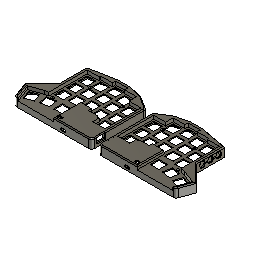
top_3x5_3 (Autodesk Fusion 360 design; units mm, degrees)
Autodesk Fusion 360 part; units mm, degrees
note: some values were not read from the file. Chosen so that the rebuilt part matches the saved one: which pieces of a blend or face edit are solid. Set by a fixed rule: which sketch regions a step uses.
sketch "case_plate_3x5_3" plane through (0, 0, 0) normal (0, 0, 1) x (1, 0, 0)
  line L0 (28.1017, -18.5688) -> (8.5, -30.9488)
  line L1 (8.5, -30.9488) -> (8.5, -112.72)
  line L2 (8.5, -112.72) -> (126.2948, -112.72)
  line L3 (133.9348, -91.7293) -> (107.5, -65.3353)
  line L4 (107.5, -65.3353) -> (107.5, -21.174)
  line L5 (126.2948, -112.72) -> (133.9348, -91.7293)
  line L6 (107.5, -21.174) -> (67.6888, -13.518)
  line L7 (67.6888, -13.518) -> (67.5953, -13.5)
  line L8 (67.5953, -13.5) -> (48.3769, -13.5)
  line L9 (48.3769, -13.5) -> (28.1017, -18.5688)
  line L10 (137.4081, -90.9579) -> (110.5, -64.0913)
  line L11 (5.5, -115.72) -> (128.3954, -115.72)
  line L12 (5.5, -29.2953) -> (5.5, -115.72)
  line L13 (110.5, -64.0913) -> (110.5, -18.6959)
  line L14 (26.9069, -15.7752) -> (5.5, -29.2953)
  line L15 (128.3954, -115.72) -> (137.4081, -90.9579)
  line L16 (110.5, -18.6959) -> (67.8811, -10.5)
  line L17 (48.0076, -10.5) -> (26.9069, -15.7752)
  line L18 (67.8811, -10.5) -> (48.0076, -10.5)
  line L19 (135.3241, -91.4207) -> (108.7, -64.8377)
  line L20 (108.7, -64.8377) -> (108.7, -20.1828)
  line L21 (127.135, -113.92) -> (135.3241, -91.4207)
  line L22 (48.2292, -12.3) -> (27.6238, -17.4513)
  line L23 (67.7096, -12.3) -> (48.2292, -12.3)
  line L24 (108.7, -20.1828) -> (67.7096, -12.3)
  line L25 (27.6238, -17.4513) -> (7.3, -30.2874)
  line L26 (7.3, -30.2874) -> (7.3, -113.92)
  line L27 (7.3, -113.92) -> (127.135, -113.92)
  line L28 (27.3848, -16.8926) -> (6.7, -29.9567)
  line L29 (136.0188, -91.2664) -> (109.3, -64.5889)
  line L30 (48.1553, -11.7) -> (27.3848, -16.8926)
  line L31 (6.7, -29.9567) -> (6.7, -114.52)
  line L32 (127.5552, -114.52) -> (136.0188, -91.2664)
  line L33 (67.7668, -11.7) -> (48.1553, -11.7)
  line L34 (109.3, -64.5889) -> (109.3, -19.6872)
  line L35 (68.0288, -11.7504) -> (67.7668, -11.7)
  line L36 (6.7, -114.52) -> (127.5552, -114.52)
  line L37 (109.3, -19.6872) -> (68.0288, -11.7504)
  circle A0 centre (32, -39.5) radius 2.2
  circle A1 centre (84, -39.5) radius 2.2
  circle A2 centre (100.1356, -83.3241) radius 2.2
  line L38 (43.5, -109.61) -> (43.5, -91.61)
  line L39 (10.5, -91.61) -> (10.5, -109.61)
  line L40 (43.5, -91.61) -> (10.5, -91.61)
  line L41 (10.5, -109.61) -> (43.5, -109.61)
  line L42 (47.025, -106.99) -> (47.025, -112.84)
  line L43 (55.825, -112.84) -> (55.825, -106.99)
  line L44 (55.825, -106.99) -> (47.025, -106.99)
  line L45 (66.825, -107.975) -> (57.825, -107.975)
  line L46 (66.825, -111.475) -> (66.825, -107.975)
  line L47 (57.825, -107.975) -> (57.825, -111.475)
  line L48 (57.825, -111.475) -> (66.825, -111.475)
  line L49 (122.6064, -82.1718) -> (114.8282, -74.3936)
  line L50 (114.8282, -74.3936) -> (108.3936, -80.8282)
  line L51 (108.3936, -80.8282) -> (110.7585, -83.1932)
  line L52 (118.9049, -85.8732) -> (122.6064, -82.1718)
  line L53 (43.2, -88.45) -> (43.2, -79.55)
  line L54 (43.2, -79.55) -> (34.7125, -79.55)
  line L55 (34.6, -79.6909) -> (34.6, -88.45)
  line L56 (34.6, -88.45) -> (43.2, -88.45)
  line L57 (27, -87) -> (27, -73)
  line L58 (13, -73) -> (13, -87)
  line L59 (13, -87) -> (27, -87)
  line L60 (27, -73) -> (13, -73)
  line L61 (27, -54) -> (13, -54)
  line L62 (27, -68) -> (27, -54)
  line L63 (13, -68) -> (27, -68)
  line L64 (13, -54) -> (13, -68)
  line L65 (13, -49) -> (27, -49)
  line L66 (13, -35) -> (13, -49)
  line L67 (27, -35) -> (13, -35)
  line L68 (27, -49) -> (27, -35)
  line L69 (32, -75) -> (46, -75)
  line L70 (46, -61) -> (32, -61)
  line L71 (32, -61) -> (32, -75)
  line L72 (46, -75) -> (46, -61)
  line L73 (32, -56) -> (46, -56)
  line L74 (46, -56) -> (46, -42)
  line L75 (32, -42) -> (32, -56)
  line L76 (46, -42) -> (32, -42)
  line L77 (46, -37) -> (46, -23)
  line L78 (32, -23) -> (32, -37)
  line L79 (32, -37) -> (46, -37)
  line L80 (46, -23) -> (32, -23)
  line L81 (65, -70) -> (65, -56)
  line L82 (65, -56) -> (51, -56)
  line L83 (51, -70) -> (65, -70)
  line L84 (51, -56) -> (51, -70)
  line L85 (51, -51) -> (65, -51)
  line L86 (65, -37) -> (51, -37)
  line L87 (65, -51) -> (65, -37)
  line L88 (51, -37) -> (51, -51)
  line L89 (51, -18) -> (51, -32)
  line L90 (65, -32) -> (65, -18)
  line L91 (65, -18) -> (51, -18)
  line L92 (51, -32) -> (65, -32)
  line L93 (84, -75) -> (84, -61)
  line L94 (70, -75) -> (84, -75)
  line L95 (84, -61) -> (70, -61)
  line L96 (70, -61) -> (70, -75)
  line L97 (84, -56) -> (84, -42)
  line L98 (70, -42) -> (70, -56)
  line L99 (70, -56) -> (84, -56)
  line L100 (84, -42) -> (70, -42)
  line L101 (70, -37) -> (84, -37)
  line L102 (70, -23) -> (70, -37)
  line L103 (84, -23) -> (70, -23)
  line L104 (84, -37) -> (84, -23)
  line L105 (89, -77.5) -> (103, -77.5)
  line L106 (103, -77.5) -> (103, -63.5)
  line L107 (103, -63.5) -> (89, -63.5)
  line L108 (89, -63.5) -> (89, -77.5)
  line L109 (89, -44.5) -> (89, -58.5)
  line L110 (103, -44.5) -> (89, -44.5)
  line L111 (89, -58.5) -> (103, -58.5)
  line L112 (103, -58.5) -> (103, -44.5)
  line L113 (89, -39.5) -> (103, -39.5)
  line L114 (89, -25.5) -> (89, -39.5)
  line L115 (103, -25.5) -> (89, -25.5)
  line L116 (103, -39.5) -> (103, -25.5)
  line L117 (84, -83.8) -> (70, -83.8)
  line L118 (70, -97.8) -> (84, -97.8)
  line L119 (70, -83.8) -> (70, -97.8)
  line L120 (84, -97.8) -> (84, -83.8)
  line L121 (90.3767, -98.3579) -> (104.164, -100.789)
  line L122 (92.8078, -84.5706) -> (90.3767, -98.3579)
  line L123 (104.164, -100.789) -> (106.5951, -87.0017)
  line L124 (106.5951, -87.0017) -> (92.8078, -84.5706)
  line L125 (123.5027, -107.234) -> (128.291, -94.0783)
  line L126 (115.1353, -89.29) -> (110.347, -102.4457)
  line L127 (110.347, -102.4457) -> (123.5027, -107.234)
  line L128 (128.291, -94.0783) -> (115.1353, -89.29)
  line L129 (8.5, -89.75) -> (29.75, -89.75)
  line L130 (29.75, -89.75) -> (29.75, -79.7)
  line L131 (10.25, -89.75) -> (10.25, -32.25)
  line L132 (29.25, -32.25) -> (10.25, -32.25)
  line L133 (48.75, -77.75) -> (48.75, -72.75)
  line L134 (48.25, -20.25) -> (29.25, -20.25)
  line L135 (29.25, -20.25) -> (29.25, -32.25)
  line L136 (48.75, -72.75) -> (67.25, -72.75)
  line L137 (67.75, -20.25) -> (67.75, -15.25)
  line L138 (67.75, -15.25) -> (48.25, -15.25)
  line L139 (48.25, -15.25) -> (48.25, -20.25)
  line L140 (67.25, -115.72) -> (67.25, -72.75)
  line L141 (86.75, -22.75) -> (86.75, -20.25)
  line L142 (86.75, -20.25) -> (67.75, -20.25)
  line L143 (105.75, -65.3353) -> (105.75, -22.75)
  line L144 (105.75, -22.75) -> (86.75, -22.75)
  line L145 (67.25, -100.55) -> (86.9722, -100.55)
  line L146 (86.9722, -100.55) -> (106.6135, -104.0133)
  line L147 (105.75, -84.0602) -> (111.608, -85.0931)
  line L148 (106.6135, -104.0133) -> (125.1463, -110.7587)
  line L149 (123.3406, -115.72) -> (131.8157, -92.4347)
  line L150 (111.7483, -85.1307) -> (133.4602, -93.0332)
  arc A3 (32, -79.7) -> (34.1857, -77.75) centre (32, -77.5) ccw
  line L151 (34.1857, -77.75) -> (48.75, -77.75)
  line L152 (107.5, -65.3353) -> (105.75, -65.3353)
  line L153 (105.75, -84.0602) -> (105.75, -65.3353)
  line L154 (8.5, -90.95) -> (30.95, -90.95)
  line L155 (35.0753, -78.95) -> (49.95, -78.95)
  line L156 (49.95, -78.95) -> (49.95, -73.95)
  line L157 (49.95, -73.95) -> (66.05, -73.95)
  line L158 (107.5, -82.5918) -> (107.5, -65.3353)
  line L159 (107.5, -82.5918) -> (110.4658, -83.1147)
  line L160 (113.7267, -83.9885) -> (133.327, -91.1224)
  line L161 (110.4658, -83.1147) -> (113.7267, -83.9885)
  line L162 (66.05, -112.72) -> (66.05, -73.95)
  line L163 (111.7483, -85.1307) -> (111.608, -85.0931)
  line L164 (32, -79.7) -> (29.75, -79.7)
  line L165 (8.5, -90.95) -> (30.95, -90.95)
  line L166 (30.95, -90.95) -> (30.95, -80.9)
  line L167 (32, -80.9) -> (30.95, -80.9)
  arc A4 (32, -80.9) -> (35.0753, -78.95) centre (32, -77.5) ccw
  line L168 (35.0753, -78.95) -> (49.95, -78.95)
  line L169 (49.95, -78.95) -> (49.95, -73.95)
  line L170 (49.95, -73.95) -> (66.05, -73.95)
  line L171 (66.05, -115.72) -> (66.05, -73.95)
  dimension "d85" = 1.2
  constraint tangent A3 L164
  constraint perpendicular L130 L164
extrude "inner-wall-down" add sketch "case_plate_3x5_3" against normal blind 6.8 contours L0 L1 L2 L3 L4 L5 L6 L7 L8 L9 L19 L20 L21 L22 L23 L24 L25 L26 L27 L149 L171 | L2 L27 L140 L171 | L2 L27 L140 L149 | L19 L20 L21 L22 L23 L24 L25 L26 L27 L28 L29 L30 L31 L32 L33 L34 L35 L36 L37 L149 L171 | L27 L36 L140 L171 | L27 L36 L140 L149 makes body 1
extrude "outer-wall-down" add sketch "case_plate_3x5_3" against normal blind 7.6 contours L10 L11 L12 L13 L14 L15 L16 L17 L18 L28 L29 L30 L31 L32 L33 L34 L35 L36 L37 L149 L171 | L11 L36 L140 L171 | L11 L36 L140 L149 bodies 1
extrude "switchplate" add sketch "case_plate_3x5_3" along normal blind 1.6 contours L129 L130 L131 L132 L133 L134 L135 L136 L137 L138 L139 L140 L141 L142 L143 L144 L145 L146 L147 L148 L149 L150 A3 L151 L153 L163 L164 | L2 L140 L145 L146 L148 L149 | L2 L27 L140 L149 | L27 L36 L140 L149 | L11 L36 L140 L149 | A0 | A1 | A2 bodies 1
extrude "raised-wall" add sketch "case_plate_3x5_3" along normal blind 7 contours L0 L1 L4 L6 L7 L8 L9 L129 L131 L132 L134 L135 L137 L138 L139 L141 L142 L143 L144 L152 | L0 L1 L2 L3 L4 L5 L6 L7 L8 L9 L19 L20 L21 L22 L23 L24 L25 L26 L27 L149 L171 | L1 L2 L45 L46 L48 L129 L130 L133 L136 L140 A3 L151 L154 L155 L156 L157 L162 L164 L165 L166 L167 A4 L168 L169 L170 L171 | L3 L5 L147 L150 L152 L153 L158 L159 L160 L161 L163 | L2 L27 L140 L171 | L45 L46 L48 L162 L171 | L19 L20 L21 L22 L23 L24 L25 L26 L27 L28 L29 L30 L31 L32 L33 L34 L35 L36 L37 L149 L171 | L27 L36 L140 L171 | L2 L5 L149 L150 | L10 L11 L12 L13 L14 L15 L16 L17 L18 L28 L29 L30 L31 L32 L33 L34 L35 L36 L37 L149 L171 | L11 L36 L140 L171 bodies 1
extrude "hollow-areas" add sketch "case_plate_3x5_3" along normal blind 1.6 from surface at 5.4 contours L1 L2 L42 L43 L44 L45 L47 L48 L53 L54 L55 L56 L154 L155 L156 L157 L162 L165 L166 L167 A4 L168 L169 L170 L171 | L2 L42 L43 L44 | L3 L49 L50 L51 L52 L158 L159 L160 L161 | L53 L54 L55 L56 A4 | L49 L50 L51 L52 L160 L161 | L45 L47 L48 L162 L171 | L38 L39 L40 L41 bodies 1
move_body "drop-to-hole-plane" bodies 1 to x (1, 0, 0) y (0, 1, 0) z (0, 0, 1) at (0, 0, -1.6)
hole "switchplate-holes" at (84, -39.5, 0) at (32, -39.5, 0) at (100.1356, -83.3241, 0) at (32, -77.5, 0) direction (0, 0, -1) diameter 2.4 end up to surface (1.6 mm away) countersink diameter 4.4 countersink angle 90 bodies 1
sketch "usb-cutout" plane through (5.5, 0, 0) normal (-1, 0, 0) x (0, -1, 0)
  line L0 (29.2953, 5.4) -> (29.2953, -9.2)
  line L1 (29.2953, -9.2) -> (115.72, -9.2)
  line L2 (115.72, -9.2) -> (115.72, 5.4)
  line L3 (115.72, 5.4) -> (29.2953, 5.4)
  line L4 (91.61, 0) -> (109.61, 0)
  line L5 (91.61, 4.2) -> (109.61, 4.2)
  line L6 (94.61, 4.2) -> (106.61, 4.2)
  line L7 (106.61, 4.2) -> (106.61, -3.8)
  line L8 (106.61, -3.8) -> (94.61, -3.8)
  line L9 (94.61, -3.8) -> (94.61, 4.2)
  point P0 (94.61, 4.2)
  point P1 (106.61, -3.8)
  dimension "d16" = 1.2
  dimension "d86" = 8
  constraint horizontal L6
  constraint vertical L7
  constraint horizontal L8
  constraint vertical L9
  constraint coincident P1 L7.end
  constraint coincident P0 L6.start
  measures "d16" distance of L3 L5
  measures "d86" distance of L5 P1
extrude "usb-cutout (1)" cut sketch "usb-cutout" against normal up to surface (3 mm away) contours L4 L5 L6 L7 L9 | L4 L7 L8 L9 bodies 1
sketch "vik-cutout" plane through (23.119, 23.1547, 0) normal (0.70656, 0.707653, 0) x (-0.707653, 0.70656, 0)
  line L0 (-161.5044, 5.4) -> (-161.5044, -9.2)
  line L1 (-161.5044, -9.2) -> (-123.48, -9.2)
  line L2 (-123.48, -9.2) -> (-123.48, 5.4)
  line L3 (-123.48, 5.4) -> (-161.5044, 5.4)
  line L4 (-144.8221, 0) -> (-133.8221, 0)
  line L5 (-144.8221, -5) -> (-133.8221, -5)
  line L6 (-142.8221, -4.5) -> (-135.8221, -4.5)
  line L7 (-135.8221, -4.5) -> (-135.8221, -5.5)
  line L8 (-135.8221, -5.5) -> (-142.8221, -5.5)
  line L9 (-142.8221, -5.5) -> (-142.8221, -4.5)
  point P0 (-142.8221, -4.5)
  point P1 (-135.8221, -5.5)
  dimension "d19" = 10.4
  constraint horizontal L6
  constraint vertical L7
  constraint horizontal L8
  constraint vertical L9
  constraint coincident P1 L7.end
  constraint coincident P0 L6.start
  measures "d19" distance of L3 L5
extrude "vik-cutout (1)" cut sketch "vik-cutout" against normal up to surface (3 mm away) contours L5 L6 L7 L9 | L5 L7 L8 L9 bodies 1
sketch "rst-cutout" plane through (0, 0, 5.4) normal (0, 0, 1) x (-1, 0, 0)
  line L0 (-131.8157, 92.4347) -> (-123.3406, 115.72)
  line L1 (-123.3406, 115.72) -> (-128.3954, 115.72)
  line L2 (-128.3954, 115.72) -> (-137.4081, 90.9579)
  line L3 (-137.4081, 90.9579) -> (-110.5, 64.0913)
  line L4 (-110.5, 64.0913) -> (-110.5, 18.6959)
  line L5 (-110.5, 18.6959) -> (-67.8811, 10.5)
  line L6 (-67.8811, 10.5) -> (-48.0076, 10.5)
  line L7 (-48.0076, 10.5) -> (-26.9069, 15.7752)
  line L8 (-26.9069, 15.7752) -> (-5.5, 29.2953)
  line L9 (-5.5, 29.2953) -> (-5.5, 115.72)
  line L10 (-5.5, 115.72) -> (-67.25, 115.72)
  line L11 (-67.25, 115.72) -> (-67.25, 72.75)
  line L12 (-57.825, 107.975) -> (-57.825, 111.475)
  line L13 (-66.825, 107.975) -> (-57.825, 107.975)
  line L14 (-66.825, 111.475) -> (-66.825, 107.975)
  line L15 (-57.825, 111.475) -> (-66.825, 111.475)
  line L16 (-59.325, 107.975) -> (-59.325, 111.475)
  line L17 (-65.325, 111.475) -> (-65.325, 107.975)
  line L18 (-105.75, 22.75) -> (-105.75, 84.0602)
  line L19 (-105.75, 84.0602) -> (-111.608, 85.0931)
  line L20 (-111.608, 85.0931) -> (-111.7483, 85.1307)
  line L21 (-111.7483, 85.1307) -> (-131.8157, 92.4347)
  line L22 (-67.25, 72.75) -> (-48.75, 72.75)
  line L23 (-48.75, 72.75) -> (-48.75, 77.75)
  line L24 (-48.75, 77.75) -> (-34.1857, 77.75)
  arc A0 (-32, 79.7) -> (-34.1857, 77.75) centre (-32, 77.5) ccw
  line L25 (-32, 79.7) -> (-29.75, 79.7)
  line L26 (-29.75, 79.7) -> (-29.75, 89.75)
  line L27 (-29.75, 89.75) -> (-10.25, 89.75)
  line L28 (-10.25, 89.75) -> (-10.25, 32.25)
  line L29 (-10.25, 32.25) -> (-29.25, 32.25)
  line L30 (-29.25, 32.25) -> (-29.25, 20.25)
  line L31 (-29.25, 20.25) -> (-48.25, 20.25)
  line L32 (-48.25, 20.25) -> (-48.25, 15.25)
  line L33 (-48.25, 15.25) -> (-67.75, 15.25)
  line L34 (-67.75, 15.25) -> (-67.75, 20.25)
  line L35 (-67.75, 20.25) -> (-86.75, 20.25)
  line L36 (-86.75, 20.25) -> (-86.75, 22.75)
  line L37 (-86.75, 22.75) -> (-105.75, 22.75)
extrude "rst-cutout (1)" cut sketch "rst-cutout" against normal up to surface (1.6 mm away) contours L13 L15 L16 L17 bodies 1
sketch "pwr-cutout" plane through (0, -115.72, 0) normal (0, -1, 0) x (1, 0, 0)
  line L0 (5.5, 5.4) -> (5.5, -9.2)
  line L1 (5.5, -9.2) -> (128.3954, -9.2)
  line L2 (128.3954, -9.2) -> (128.3954, 5.4)
  line L3 (128.3954, 5.4) -> (123.3406, 5.4)
  line L4 (123.3406, 5.4) -> (123.3406, 0)
  line L5 (123.3406, 0) -> (67.25, 0)
  line L6 (67.25, 0) -> (67.25, 5.4)
  line L7 (67.25, 5.4) -> (5.5, 5.4)
  line L8 (55.825, 0) -> (47.025, 0)
  line L9 (55.825, -5) -> (47.025, -5)
  line L10 (49.425, -5.75) -> (53.425, -5.75)
  arc A0 (53.425, -5.75) -> (53.425, -2.75) centre (53.425, -4.25) ccw
  line L11 (53.425, -2.75) -> (49.425, -2.75)
  arc A1 (49.425, -2.75) -> (49.425, -5.75) centre (49.425, -4.25) ccw
  line L12 (49.425, -4.25) -> (53.425, -4.25) construction
  point P0 (49.425, -4.25)
  point P1 (53.425, -4.25)
  dimension "d24" = 10.4
  dimension "d25" = 3
  constraint tangent L10 A0
  constraint tangent A0 L11
  constraint parallel L10 L11
  constraint tangent L11 A1
  constraint tangent L10 A1
  constraint coincident P1 A0.centre
  constraint parallel L9 L12
  constraint coincident P0 A1.centre
  measures "d24" distance of L7 L9
  measures "d25" diameter of A0
extrude "pwr-cutout (1)" cut sketch "pwr-cutout" against normal up to surface (3 mm away) contours L9 L10 A0 A1 | L9 A0 L11 A1 bodies 1
sketch "pwr-tab-slot" plane through (0, 0, -5.75) normal (0, 0, 1) x (-1, 0, 0)
  line L0 (-49.425, 115.72) -> (-53.425, 115.72)
  line L1 (-53.425, 115.72) -> (-53.425, 112.72)
  line L2 (-53.425, 112.72) -> (-49.425, 112.72)
  line L3 (-49.425, 112.72) -> (-49.425, 115.72)
  line L4 (-49.425, 114.22) -> (-53.425, 114.22)
  dimension "d28" = 1.5
  constraint coincident L3 L4.start
  constraint coincident L1 L4.end
  constraint perpendicular L1 L4
  measures "d28" distance of L2 L4
extrude "pwr-tab-slot (1)" cut sketch "pwr-tab-slot" against normal up to surface (2.65 mm away) contours L1 L2 L3 L4 bodies 1
sketch "Sketch11" plane through (110.5, 0, 0) normal (1, 0, 0) x (0, 1, 0)
  line L0 (-64.0913, 5.4) -> (-64.0913, -9.2)
  line L1 (-64.0913, -9.2) -> (-18.6959, -9.2)
  line L2 (-18.6959, -9.2) -> (-18.6959, 5.4)
  line L3 (-18.6959, 5.4) -> (-64.0913, 5.4)
  line L4 (-64.0913, -1.5) -> (-18.6959, -1.5) construction
  line L5 (-54.3936, -2.25) -> (-28.3936, -2.25)
  arc A0 (-28.3936, -2.25) -> (-28.3936, -0.75) centre (-28.3936, -1.5) ccw
  line L6 (-28.3936, -0.75) -> (-54.3936, -0.75)
  arc A1 (-54.3936, -0.75) -> (-54.3936, -2.25) centre (-54.3936, -1.5) ccw
  line L7 (-54.3936, -1.5) -> (-28.3936, -1.5) construction
  line L8 (-52.1203, 2.4874) -> (-56.7102, 2.4625)
  line L9 (-56.7102, 2.4625) -> (-58.9835, -1.5249)
  line L10 (-58.9835, -1.5249) -> (-56.667, -5.4874)
  line L11 (-56.667, -5.4874) -> (-52.0771, -5.4625)
  line L12 (-52.0771, -5.4625) -> (-49.8038, -1.4751)
  line L13 (-49.8038, -1.4751) -> (-52.1203, 2.4874)
  line L14 (-39.1203, 2.4874) -> (-43.7102, 2.4625)
  line L15 (-43.7102, 2.4625) -> (-45.9835, -1.5249)
  line L16 (-45.9835, -1.5249) -> (-43.667, -5.4874)
  line L17 (-43.667, -5.4874) -> (-39.0771, -5.4625)
  line L18 (-39.0771, -5.4625) -> (-36.8038, -1.4751)
  line L19 (-36.8038, -1.4751) -> (-39.1203, 2.4874)
  line L20 (-26.1203, 2.4874) -> (-30.7102, 2.4625)
  line L21 (-30.7102, 2.4625) -> (-32.9835, -1.5249)
  line L22 (-32.9835, -1.5249) -> (-30.667, -5.4874)
  line L23 (-30.667, -5.4874) -> (-26.0771, -5.4625)
  line L24 (-26.0771, -5.4625) -> (-23.8038, -1.4751)
  line L25 (-23.8038, -1.4751) -> (-26.1203, 2.4874)
  point P0 (-41.3936, -1.5)
  point P1 (-28.3936, -1.5)
  point P2 (-54.3936, -1.5)
  point P3 (-54.3936, -1.5)
  point P4 (-41.3936, -1.5)
  point P5 (-28.3936, -1.5)
  point P6 (-54.3936, -1.5)
  point P7 (-41.3936, -1.5)
  point P8 (-28.3936, -1.5)
  dimension "d89" = 6.9
  dimension "d90" = 13
  dimension "d91" = 13
  dimension "d95" = 1.5
  dimension "d109" = 3.975
  dimension "d110" = 3.975
  dimension "d111" = 3.975
  constraint coincident L0 L4.start
  constraint coincident L2 L4.end
  constraint perpendicular L2 L4
  constraint coincident L4 P4
  constraint midpoint L4 P4
  constraint coincident L4 P5
  constraint coincident L4 P6
  constraint coincident P6 P3
  constraint coincident P4 P0
  constraint coincident P5 P1
  constraint tangent L5 A0
  constraint tangent A0 L6
  constraint parallel L5 L6
  constraint tangent L6 A1
  constraint tangent L5 A1
  measures "d89" distance of L3 L4
  measures "d90" distance of P4 P6
  measures "d91" distance of P4 P5
  measures "d95" diameter of A0
  measures "d109" distance of P6 L13
  measures "d110" distance of P7 L19
  measures "d111" distance of P8 L25
sketch "Sketch12" plane through (23.119, 23.1547, 0) normal (0.70656, 0.707653, 0) x (-0.707653, 0.70656, 0)
  line L0 (-142.8221, -5.5) -> (-142.8221, -4.5)
  line L1 (-142.8221, -4.5) -> (-135.8221, -4.5)
  line L2 (-135.8221, -4.5) -> (-135.8221, -5.5)
  line L3 (-135.8221, -5.5) -> (-142.8221, -5.5)
  line L4 (-161.5044, 5.4) -> (-161.5044, -9.2)
  line L5 (-161.5044, -9.2) -> (-123.48, -9.2)
  line L6 (-123.48, -9.2) -> (-123.48, 5.4)
  line L7 (-123.48, 5.4) -> (-161.5044, 5.4)
  line L8 (-123.48, -1.5) -> (-161.5044, -1.5) construction
  line L9 (-149.5044, -2.25) -> (-131.48, -2.25)
  arc A0 (-131.48, -2.25) -> (-131.48, -0.75) centre (-131.48, -1.5) ccw
  line L10 (-131.48, -0.75) -> (-149.5044, -0.75)
  arc A1 (-149.5044, -0.75) -> (-149.5044, -2.25) centre (-149.5044, -1.5) ccw
  line L11 (-149.5044, -1.5) -> (-131.48, -1.5) construction
  line L12 (-129.1853, 2.4751) -> (-133.7752, 2.4749)
  line L13 (-133.7752, 2.4749) -> (-136.07, -1.5003)
  line L14 (-136.07, -1.5003) -> (-133.7748, -5.4751)
  line L15 (-133.7748, -5.4751) -> (-129.1848, -5.4749)
  line L16 (-129.1848, -5.4749) -> (-126.8901, -1.4997)
  line L17 (-126.8901, -1.4997) -> (-129.1853, 2.4751)
  line L18 (-147.1962, 2.4673) -> (-151.7862, 2.4826)
  line L19 (-151.7862, 2.4826) -> (-154.0943, -1.4847)
  line L20 (-154.0943, -1.4847) -> (-151.8126, -5.4673)
  line L21 (-151.8126, -5.4673) -> (-147.2227, -5.4826)
  line L22 (-147.2227, -5.4826) -> (-144.9145, -1.5153)
  line L23 (-144.9145, -1.5153) -> (-147.1962, 2.4673)
  point P0 (-149.5044, -1.5)
  point P1 (-131.48, -1.5)
  point P2 (-149.5044, -1.5)
  point P3 (-131.48, -1.5)
  point P4 (-131.48, -1.5)
  point P5 (-149.5044, -1.5)
  dimension "d96" = 6.9
  dimension "d97" = 8
  dimension "d98" = 12
  dimension "d101" = 1.5
  dimension "d107" = 3.975
  dimension "d108" = 3.975
  constraint coincident L6 L8.start
  constraint coincident L4 L8.end
  constraint perpendicular L4 L8
  constraint coincident L8 P5
  constraint coincident L8 P4
  constraint coincident P5 P2
  constraint coincident P4 P3
  constraint tangent L9 A0
  constraint tangent A0 L10
  constraint parallel L9 L10
  constraint tangent L10 A1
  constraint tangent L9 A1
  constraint parallel L8 L11
  measures "d96" distance of L7 L8
  measures "d97" distance of L8.start P4
  measures "d98" distance of L4 P5
  measures "d101" diameter of A0
  measures "d107" distance of P4 L17
  measures "d108" distance of P5 L23
extrude "Extrude20" cut sketch "Sketch12" against normal blind 2 contours L9 L10 A1 L22 L23 | L9 L10 A1 L18 L19 L20 L21 L22 L23 | L9 L10 L13 L14 L22 L23 | L9 A0 L10 L13 L14 | L9 A0 L10 L12 L13 L14 L15 L16 L17 bodies 1
extrude "Extrude21" cut sketch "Sketch11" against normal blind 2 contours L5 L6 A1 L12 L13 | L5 L6 A1 L8 L9 L10 L11 L12 L13 | L5 L6 L12 L13 L15 L16 | L5 L6 L15 L16 L18 L19 | L5 L16 L17 L18 | L5 L6 L18 L19 L21 L22 | L6 L14 L15 L19 | L5 A0 L6 L21 L22 | L5 A0 L6 L20 L21 L22 L23 L24 L25 bodies 1
chamfer "Chamfer6" distance 0.4 angle 45 30 edges at (110.5, -28.372, -5.4749) (110.5, -24.9404, -3.4688) (110.5, -24.962, 0.5062) (110.5, -28.4152, 2.4749) (110.5, -31.6259, 0.8562) (110.5, -31.6133, -3.8687) (110.5, -38.1613, -3.8562) (110.5, -38.174, 0.8687) (110.5, -41.4152, 2.4749) (110.5, -44.6259, 0.8562) (110.5, -44.6133, -3.8687) (110.5, -41.372, -5.4749) (110.5, -51.174, 0.8687) (110.5, -51.1613, -3.8562) (110.5, -54.4152, 2.4749) (110.5, -57.8468, 0.4688) (110.5, -57.8252, -3.5062) (110.5, -54.372, -5.4749) (128.9069, -82.4698, 2.475) (131.3476, -84.9067, 0.499) (131.357, -84.9161, -3.476) (128.9256, -82.4885, -5.475) (126.6306, -80.1971, 0.8587) (126.6361, -80.2025, -3.8663) (118.4441, -72.0232, 0.8624) (116.1614, -69.744, 2.475) (118.444, -72.0231, -3.8626) (116.1611, -69.7437, -5.475) (113.7252, -67.3116, 0.4877) (113.7251, -67.3114, -3.4873) on bodies 1
fillet "Fillet1" radius 5 15 edges at (67.8811, -10.5, -1.9) (48.0076, -10.5, -1.9) (26.9069, -15.7752, -1.9) (5.5, -29.2953, -1.9) (5.5, -115.72, -1.9) (128.3954, -115.72, -1.9) (127.5552, -114.52, -8.8) (6.7, -114.52, -8.8) (6.7, -29.9567, -8.8) (27.3848, -16.8926, -8.8) (28.1017, -18.5688, -5) (48.1553, -11.7, -8.8) (48.3769, -13.5, -5) (67.5953, -13.5, -5) (67.7668, -11.7, -8.8) on bodies 1
fillet "Fillet1" radius 2 3 edges at (126.2948, -112.72, -5) (8.5, -112.72, -2.3) (8.5, -30.9488, -5) on bodies 1
chamfer "top-edge" distance 1.5 angle 45 18 edges at (124.1175, -115.72, 5.4) (127.7623, -114.8157, 5.4) (133.5005, -101.694, 5.4) (123.954, -77.5246, 5.4) (38.875, -115.72, 5.4) (6.9645, -114.2555, 5.4) (5.5, -71.3856, 5.4) (6.1211, -29.6376, 5.4) (17.0292, -22.0137, 5.4) (26.9321, -15.834, 5.4) (37.548, -13.1149, 5.4) (48.0122, -10.5375, 5.4) (58.0139, -10.5, 5.4) (67.879, -10.5225, 5.4) (89.4245, -14.643, 5.4) (110.5, -41.3936, 5.4) (67.25, -94.235, 5.4) (127.5781, -104.0773, 5.4) on bodies 1
chamfer "rst" distance 0.4 angle 45 4 edges at (62.325, -107.975, 5.4) (59.325, -109.725, 5.4) (62.325, -111.475, 5.4) (65.325, -109.725, 5.4) on bodies 1
chamfer "pwr" distance 0.5 angle 45 4 edges at (51.425, -115.72, -2.75) (54.925, -115.72, -4.25) (51.425, -115.72, -5.75) (47.925, -115.72, -4.25) on bodies 1
chamfer "usb" distance 1 angle 45 3 edges at (5.5, -94.61, 0.2) (5.5, -100.61, -3.8) (5.5, -106.61, 0.2) on bodies 1
mirror "Mirror1" about plane through (0, 0, 0) normal (1, 0, 0) of bodies 1 makes body 2
